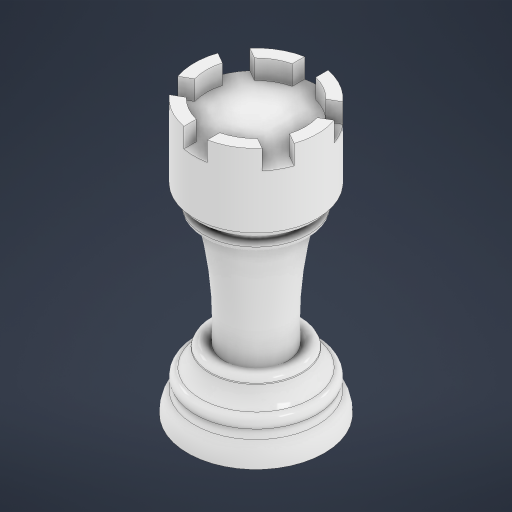
# Autodesk Inventor part: věž bílá
Saved by Autodesk Inventor 2023 (Build 270158000, 158)
## iProperties
Created: 2023-04-20
Part Number: věž bílá
Material: Generic
Document SubType Name: Modeling
Designer: 19LBoreckyP
Density: 1 g/cm^3
Appearance: Default
Author: 19LBoreckyP
Autodesk Inventor part; units mm, degrees
ref_plane "YZ Plane" through (0, 0, 0) normal (1, 0, 0) x (0, 1, 0)
ref_plane "XZ Plane" through (0, 0, 0) normal (0, 1, 0) x (-1, 0, 0)
ref_plane "XY Plane" through (0, 0, 0) normal (0, 0, 1) x (1, 0, 0)
sketch "Sketch1" plane through (0, 0, 0) normal (0, 0, 1) x (1, 0, 0)
  arc A0 (98.2828, 24.0196) -> (100.6664, 19.59) centre (106.749, 25.7193) ccw
  arc A1 (102.0066, 16.7545) -> (100.6664, 19.59) centre (100.2382, 17.6531) ccw
  arc A2 (103.989, 9.2026) -> (102.2375, 14.5873) centre (96.1287, 9.6232) ccw
  arc A3 (102.0066, 16.7545) -> (102.2375, 14.5873) centre (103.7897, 15.8486) ccw
  line L0 (86.489, 9.2026) -> (86.489, 79.2026) construction
  line L1 (86.489, 9.2026) -> (156.489, 9.2026) construction
  line L2 (102.2471, 60.4536) -> (102.2471, 79.2026)
  line L3 (102.2471, 79.2026) -> (99.1423, 79.2026)
  line L4 (99.1423, 79.2026) -> (99.1423, 74.2026)
  line L5 (99.1423, 74.2026) -> (86.489, 74.2026)
  arc A4 (98.5312, 58.3956) -> (101.6196, 60.4536) centre (99.3797, 60.4687) ccw
  arc A5 (99.9633, 55.6846) -> (97.9367, 56.2648) centre (98.8586, 55.6556) ccw
  arc A6 (97.551, 54.7786) -> (99.9633, 55.6846) centre (98.6004, 55.6488) ccw
  arc A7 (98.5312, 58.3956) -> (97.9367, 56.2648) centre (197.2889, 29.6902) ccw
  arc A8 (97.551, 54.7786) -> (94.5556, 24.9017) centre (197.2889, 29.6902) ccw
  arc A9 (98.2213, 24.2546) -> (94.5556, 24.9017) centre (96.2166, 23.6048) ccw
  line L6 (101.6196, 60.4536) -> (102.2471, 60.4536)
  arc A10 (98.2828, 24.0196) -> (98.2213, 24.2546) centre (97.4401, 23.9248) ccw
  line L7 (86.489, 74.2026) -> (86.489, 9.2026)
  line L8 (86.489, 9.2026) -> (103.989, 9.2026)
  dimension "d0" = 2
  dimension "d3" = 70
  dimension "d4" = 90
  dimension "d5" = 5
  constraints: 22 point on circle, 18 end point, 11 centre point, 4 perpendicular, 3 tangent, 2 collinear, 2 horizontal, 1 point on line, 1 vertical
  measures "d0" radius of A3
  measures "d3" distance of L0.start L0.end
  measures "d4" angle of L1 L0
  measures "d5" distance of L3.end L4.end
revolve "Revolution1" add sketch "Sketch1" angle 360 about axis through (86.489, 9.2026, 0) along (0, 1, 0)
ref_plane "Work Plane4" through (86.489, 74.2026, 0) normal (0, -1, 0) x (1, 0, 0)
sketch "Sketch2" plane through (86.489, 74.2026, 0) normal (0, -1, 0) x (1, 0, 0)
  circle A0 centre (0, 0) radius 12.6533 projected
  circle A1 centre (0, 0) radius 15.7475 projected
  line L0 (-3.0004, -15.7475) -> (-3.0004, 24.2525)
  line L1 (-3.0004, -15.7475) -> (36.9996, -15.7475) construction
  line L2 (-3.0004, 24.2525) -> (-0.0004, 24.2525)
  line L3 (-0.0004, 24.2525) -> (2.9996, 24.2525)
  line L4 (2.9996, 24.2525) -> (2.9996, -15.7475)
  line L5 (0, 0) -> (21.9162, -12.6533)
  line L6 (0, 0) -> (25.3066, 0) construction
  line L7 (0, 0) -> (-24.2755, 14.0154)
  line L8 (12.0261, -10.4041) -> (-25.774, 11.4198)
  line L9 (-25.774, 11.4198) -> (-22.7755, 16.6135)
  line L10 (-22.7755, 16.6135) -> (15.1377, -5.2756)
  line L11 (0, 0) -> (25.661, 14.8154)
  line L12 (0, 0) -> (29.6308, 0) construction
  line L13 (25.661, 14.8154) -> (27.161, 12.2173)
  line L14 (25.661, 14.8154) -> (24.161, 17.4135)
  line L15 (24.161, 17.4135) -> (-22.7755, -9.6853)
  line L16 (-22.7755, -9.6853) -> (-19.7755, -14.8815)
  line L17 (-19.7755, -14.8815) -> (27.161, 12.2173)
  line L18 (-3.0004, -15.7475) -> (-3.0004, -19.4076)
  line L19 (-3.0004, -19.4076) -> (2.9996, -19.4076)
  line L20 (2.9996, -19.4076) -> (2.9996, -15.7475)
  line L21 (12.0261, -10.4041) -> (14.9419, -12.0923)
  line L22 (14.9419, -12.0923) -> (17.9426, -6.895)
  line L23 (17.9426, -6.895) -> (15.1377, -5.2756)
  point P0 (-86.489, 0)
  point P1 (-5.9972, 0.0016)
  point P2 (-3.0004, -5.1964)
  point P3 (2.9996, -5.1926)
  point P4 (6, 0)
  point P5 (2.9996, 5.1959)
  point P6 (-3.0004, 5.1964)
  dimension "d10" = 40
  dimension "d11" = 90
  dimension "d12" = 3
  dimension "d13" = 3
  dimension "d14" = 30
  dimension "d17" = 30
  dimension "d18" = 3
  dimension "d19" = 3
  dimension "d20" = 6
  constraints: 48 end point, 10 perpendicular, 3 equal length, 3 horizontal, 2 point on line, 1 vertical
  measures "d10" distance of L0.start L0.end
  measures "d11" angle of L1 L0
  measures "d12" distance of L0.end L2.end
  measures "d13" distance of L2.end L3.end
  measures "d14" angle of L5 L6
  measures "d17" angle of L12 L11
  measures "d18" distance of L11.end L13.end
  measures "d19" distance of L11.end L14.end
  measures "d20" distance of L15.end L16.end
extrude "Extrusion1" cut sketch "Sketch2" against normal blind 10 contours L17 L10 L11 A0 | A0 L11 A1 L17 | L10 A1 L5 A0 | A0 L5 L17 L10 | L11 L4 L15 A0 | A0 L15 A1 L11 | L17 L4 L10 | A1 L11 L13 L17 | L5 A1 L8 A0 | A0 L8 L4 L5 | L10 L23 L22 L5 A1 | L10 L15 L4 | L11 L7 L15 L10 | L4 L5 L11 | A1 L15 L14 L11 | L17 L8 L0 L7 L5 | L4 L8 L17 | L5 L22 L21 L8 A1 | L4 L15 L10 L0 A0 | A0 L0 A1 L4 | L15 L0 L10 | L4 A0 L0 L17 L8 | L17 L0 L8 | L4 A1 L0 A0 | A1 L0 L2 L3 L4 | L0 L7 A0 L10 | L15 L8 A0 L7 | L0 L8 L15 | L0 L17 A0 L15 L8 | L4 L20 L19 L18 L0 A1 | A0 L7 A1 L10 | A0 L8 A1 L7 | L17 A1 L15 A0 | A1 L7 L9 L10 | A1 L8 L9 L7 | L17 L16 L15 A1
